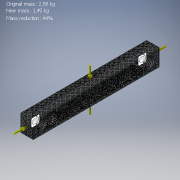
# Autodesk Inventor part: ejemplo_tibia
Saved by Autodesk Inventor 2018.3 (Build 223284000, 284)
## iProperties
Created: 2019-02-07
Part Number: ejemplo_tibia
Material: Generic
Document SubType Name: Modeling
Designer: vigus
Mass: 328.768 g
Surface Area: 471.635 cm^2
Volume: 328.768 cm^3
Density: 1 g/cm^3
Appearance: Default
Author: vigus
Autodesk Inventor part; units mm, degrees
ref_plane "YZ Plane" through (0, 0, 0) normal (1, 0, 0) x (0, 1, 0)
ref_plane "XZ Plane" through (0, 0, 0) normal (0, 1, 0) x (-1, 0, 0)
ref_plane "XY Plane" through (0, 0, 0) normal (0, 0, 1) x (1, 0, 0)
sketch "Sketch1" plane through (0, 0, 0) normal (1, 0, 0) x (0, 1, 0)
  line L0 (12.0042, 143.7964) -> (-27.9958, 143.7964)
  line L1 (-27.9958, 143.7964) -> (-27.9958, -156.2036)
  line L2 (-27.9958, -156.2036) -> (12.0042, -156.2036)
  line L3 (12.0042, -156.2036) -> (12.0042, 143.7964)
  point P0 (0, 0)
  dimension "d0" = 300
  dimension "d1" = 40
  constraints: 8 end point, 2 parallel, 1 horizontal, 1 perpendicular
  measures "d0" distance between parallel lines of L2 L0
  measures "d1" distance between parallel lines of L1 L3
extrude "Extrusion1" add sketch "Sketch1" along normal blind 30
sketch "Sketch2" plane through (30, 0, 0) normal (1, 0, 0) x (0, 0, -1)
  circle A0 centre (-123.621, -6.7738) radius 12.1593
  circle A1 centre (130.9593, -6.7738) radius 13.5475
  point P0 (0, 0)
  constraints: 2 centre point
extrude "Extrusion2" cut sketch "Sketch2" against normal blind 30
body "Solid1"
